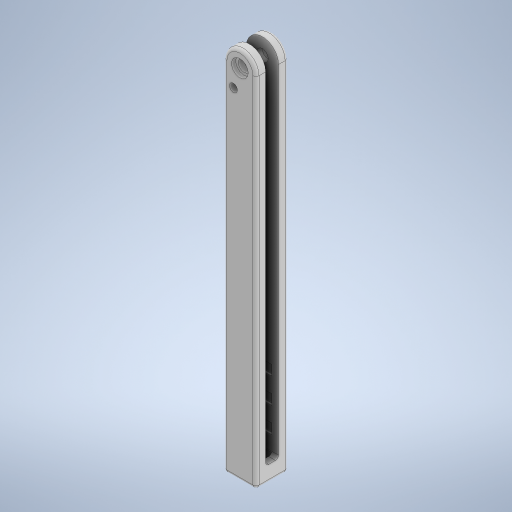
# Autodesk Inventor part: Body
Saved by Autodesk Inventor 2023.5 (Build 275446000, 446)
## iProperties
Created: 2025-04-01
Part Number: Body
Material: Generic
Document SubType Name: Modeling
Designer: huy20
Density: 1 g/cm^3
Appearance: Default
Author: huy20
Autodesk Inventor part; units mm, degrees
ref_plane "YZ Plane" through (0, 0, 0) normal (1, 0, 0) x (0, 1, 0)
ref_plane "XZ Plane" through (0, 0, 0) normal (0, 1, 0) x (-1, 0, 0)
ref_plane "XY Plane" through (0, 0, 0) normal (0, 0, 1) x (1, 0, 0)
sketch "Sketch1" plane through (0, 0, 0) normal (0, 0, 1) x (1, 0, 0)
  line L0 (6.35, 70.485) -> (6.35, -70.485)
  line L1 (6.35, -70.485) -> (-6.35, -70.485)
  line L2 (-6.35, -70.485) -> (-6.35, 70.485)
  line L3 (-6.35, 70.485) -> (6.35, -70.485) construction
  line L4 (6.35, 70.485) -> (-6.35, -70.485) construction
  arc A0 (6.2478, 69.3501) -> (-6.2478, 69.3501) centre (0, 70.485) ccw
  circle A1 centre (0, 70.485) radius 2.286
  point P0 (0, 0)
  point P1 (-6.35, 70.485)
  dimension "d0" = 12.7
  dimension "d1" = 140.97
  dimension "d2" = 4.572
  constraints: 10 end point, 3 point on circle, 2 centre point, 2 midpoint, 2 point on line, 2 tangent, 1 coincident, 1 horizontal, 1 parallel, 1 vertical
  measures "d0" distance between parallel lines of L2 L0
  measures "d1" distance of L0.start L0.end
  measures "d2" diameter of A1
extrude "Extrusion1" add sketch "Sketch1" along normal mid plane 12.7
sketch "Sketch2" plane through (6.35, -70.485, 6.35) normal (1, 0, 0) x (0, 0, -1)
  line L0 (3.81, 6.35) -> (8.89, 6.35)
  line L1 (8.89, 6.35) -> (8.89, 126.398)
  line L2 (8.89, 126.398) -> (3.81, 126.398)
  line L3 (3.81, 126.398) -> (3.81, 6.35)
  line L4 (3.81, 6.35) -> (8.89, 126.398) construction
  line L5 (8.89, 6.35) -> (3.81, 126.398) construction
  line L6 (0, 0) -> (12.7, 0) projected
  line L7 (12.7, 140.97) -> (12.7, 0) projected
  line L8 (3.81, 126.398) -> (8.89, 126.398)
  line L9 (8.89, 126.398) -> (8.89, 150.398)
  line L10 (8.89, 150.398) -> (3.81, 150.398)
  line L11 (3.81, 150.398) -> (3.81, 126.398)
  point P0 (6.35, 70.485)
  point P1 (6.35, 66.374)
  dimension "d5" = 6.35
  dimension "d6" = 5.08
  dimension "d7" = 3.81
  dimension "d8" = 120.048
  dimension "d9" = 5.08
  dimension "d10" = 24
  constraints: 20 end point, 4 parallel, 2 horizontal, 2 midpoint, 2 perpendicular
  measures "d5" distance between parallel lines of L6 L0
  measures "d6" distance between parallel lines of L3 L1
  measures "d7" distance between parallel lines of L7 L1
  measures "d8" distance of L0.end L1.end
  measures "d9" distance of L9.end L10.end
  measures "d10" distance of L8.end L9.end
extrude "Extrusion2" cut sketch "Sketch2" against normal blind 8.89 contours L3 L2 L1 L0
extrude "Extrusion3" cut sketch "Sketch2" against normal through all contours L11 L10 L9 L2
sketch "Sketch3" plane through (0, 0, 6.35) normal (0, 0, 1) x (1, 0, 0)
  circle A0 centre (0, 70.485) radius 2.286 projected
  circle A1 centre (-2.54, 62.531) radius 1.5875
  point P0 (0, 0)
  dimension "d15" = 3.175
  dimension "d16" = 7.954
  dimension "d17" = 2.54
  constraints: 1 centre point
  measures "d15" diameter of A1
  measures "d16" vertical distance of A0.centre A1.centre
  measures "d17" horizontal distance of A0.centre A1.centre
extrude "Extrusion4" cut sketch "Sketch3" against normal through all contours A1
fillet "Fillet1" radius 1.2 14 edges at (-4.445, 55.913, -2.54) (-4.445, 55.913, 2.54) (0, 76.835, 6.35) (-6.35, 0, 6.35) (6.35, 0, 6.35) (0, 76.835, -6.35) (-6.35, 0, -6.35) (6.35, 0, -6.35) (6.35, -70.485, 0) (0, -70.485, 6.35) (-6.35, -70.485, 0) (0, -70.485, -6.35) (1.905, -64.135, -2.54) (1.905, -64.135, 2.54)
sketch "Sketch5" plane through (0, 0, 6.35) normal (0, 0, 1) x (1, 0, 0)
  circle A0 centre (0, 70.485) radius 2.286 projected
  circle A1 centre (0, 70.485) radius 3.302
  point P0 (0, 0)
  dimension "d25" = 6.604
  constraints: 1 centre point, 1 coincident
  measures "d25" diameter of A1
extrude "Extrusion6" cut sketch "Sketch5" against normal blind 1.651
ref_plane "Work Plane1" through (0, 0, 0) normal (0, 0, 1) x (1, 0, 0)
mirror "Mirror1" about plane through (0, 0, 0) normal (0, 0, 1) of "Extrusion6"
sketch "Sketch6" plane through (-6.35, -69.285, 5.15) normal (-1, 0, 0) x (0, 0, 1)
  line L0 (0, 139.77) -> (0, 0) projected
  line L1 (-2.61, 139.77) -> (0, 139.77) projected
  line L2 (-2.61, 139.77) -> (-2.61, 126.398) projected
  arc A0 (-3.81, 125.198) -> (-2.61, 126.398) centre (-3.81, 126.398) ccw projected
  line L3 (-3.81, 125.198) -> (-6.49, 125.198) projected
  arc A1 (-7.69, 126.398) -> (-6.49, 125.198) centre (-6.49, 126.398) ccw projected
  line L4 (-7.69, 126.398) -> (-7.69, 139.77) projected
  line L5 (-10.3, 139.77) -> (-7.69, 139.77) projected
  line L6 (-10.3, 0) -> (-10.3, 139.77) projected
  line L7 (0, 0) -> (-10.3, 0) projected
  line L8 (-1.5, 2) -> (-8.5, 2)
  line L9 (-8.5, 2) -> (-8.5, 6)
  line L10 (-8.5, 6) -> (-1.5, 6)
  line L11 (-1.5, 6) -> (-1.5, 2)
  line L12 (-8.5, 16) -> (-1.5, 16)
  line L13 (-8.5, 12) -> (-8.5, 16)
  line L14 (-1.5, 12) -> (-8.5, 12)
  line L15 (-1.5, 16) -> (-1.5, 12)
  line L16 (-8.5, 26) -> (-1.5, 26)
  line L17 (-8.5, 22) -> (-8.5, 26)
  line L18 (-1.5, 22) -> (-8.5, 22)
  line L19 (-1.5, 26) -> (-1.5, 22)
  line L20 (-8.5, 36) -> (-1.5, 36)
  line L21 (-8.5, 32) -> (-8.5, 36)
  line L22 (-1.5, 32) -> (-8.5, 32)
  line L23 (-1.5, 36) -> (-1.5, 32)
  point P0 (-5.15, 69.285)
  dimension "d28" = 1.5
  dimension "d29" = 2
  dimension "d30" = 7
  dimension "d31" = 4
  dimension "d37" = 10
  constraints: 32 end point, 2 parallel, 1 collinear, 1 horizontal, 1 perpendicular, 1 vertical, 23 other
  measures "d28" distance between parallel lines of L0 L11
  measures "d29" distance between parallel lines of L7 L8
  measures "d30" distance of L9.end L10.end
  measures "d31" distance of L10.end L8.start
  measures "d37" distance of L9.end L12.start
extrude "Extrusion7" cut sketch "Sketch6" against normal blind 10 contours L8 L9 L10 L11 | L12 L15 L14 L13 | L16 L19 L18 L17 | L20 L23 L22 L21
body "Solid1"
